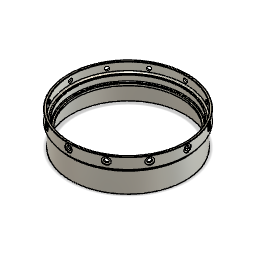
Connection-Ring-female-21.10.2024 v13 (Autodesk Fusion 360 design; units mm, degrees)
Autodesk Fusion 360 part; units mm, degrees
sketch "Skizze1" plane through (0, 0, 0) normal (0, 0, 1) x (1, 0, 0)
  line L0 (-83, 47) -> (-83, 30)
  line L1 (-83, 30) -> (-80, 30)
  line L2 (-80, 30) -> (-80, 0)
  line L3 (-73, 22.5) -> (-73, 25.5)
  line L4 (-73, 25.5) -> (-76, 25.5)
  line L5 (-76, 25.5) -> (-76, 34)
  line L6 (-76, 34) -> (-80, 34)
  line L7 (-80, 34) -> (-80, 47)
  line L8 (-80, 47) -> (-83, 47)
  line L9 (-80, 0) -> (-79, 0)
  line L10 (-76.75, 22.5) -> (-73, 22.5)
  line L11 (-76.75, 22.5) -> (-79, 0)
  line L12 (-76, 30) -> (-76.75, 22.5)
  dimension "d2" = 3
  dimension "d6" = 13
  dimension "d7" = 80
  dimension "d8" = 3
  dimension "d9" = 4
  dimension "d10" = 3
  dimension "d21" = 4
  dimension "d22" = 8.5
  dimension "d23" = 3
  dimension "d24" = 30
  dimension "d25" = 1
  constraint vertical L0
  constraint perpendicular L0 L1
  constraint perpendicular L1 L2
  constraint perpendicular L2 L4
  constraint perpendicular L5 L6
  constraint perpendicular L6 L7
  constraint perpendicular L0 L8
  constraint perpendicular L2 L9
  constraint horizontal origin L2.end
  constraint coincident L5 L12.start
  constraint collinear L11 L12
  constraint horizontal L1.end L12.start
  measures "d2" distance of L3 L5
  measures "d6" distance of L6 L8
  measures "d7" distance of origin L2
  measures "d8" distance of L0 L7
  measures "d9" distance of L2 L5
  measures "d10" distance of L0 L2
  measures "d21" distance of L1 L6
  measures "d22" distance of L4 L6
  measures "d23" distance of L4 L10
  measures "d24" distance of L1 L9
  measures "d25" distance of L2.end L9.end
revolve "Drehen1" add sketch "Skizze1" angle 360 about axis through (0, 1.75, 0) along (0, 1, 0)
fillet "Abrundung1" radius 2 1 edges at (-77.3832, 30, 30.0141)
fillet "Abrundung2" radius 2 1 edges at (-74.5862, 30, 28.9292)
fillet "Abrundung3" radius 2 1 edges at (-74.5862, 34, 28.9292)
chamfer "Fase3" distance 1 angle 45 1 edges at (-70.8569, 25.5, 27.4828)
ref_plane "Arbeitsebene1" through (83, 38.5, 0) normal (1, 0, 0) x (0, 0, -1)
sketch "Skizze4" plane through (83, 0, 0) normal (1, 0, 0) x (0, 0, -1)
  line L0 (-82.5, 47) -> (82.5, 47)
  point P0 (0, 40.5)
  dimension "d34" = 6.5
  constraint vertical origin P0
  measures "d34" distance of P0 L0
hole "Bohrung2" at (83, 40.5, 0) direction (-1, 0, 0) diameter 5.5 depth 16 tip angle 118 counterbore diameter 10 counterbore depth 1
pattern_circular "C-Anordnung1" count 12 over 360 about axis through (0, 1.75, 0) along (0, 1, 0) of "Bohrung2"
chamfer "Fase4" distance 0.4 angle 45 7 edges at (-74.5862, 47, 28.9292) (-70.8569, 34, 27.4828) (-74.5862, 0, 28.9292) (-73.6539, 0, 28.5676) (-71.5561, 22.5, 27.754) (-68.0599, 22.5, 26.3979) (-77.3832, 47, 30.0141)
equation "d7 = ( 160 / 2 ) * 1 mm"
equation "d22 = 15 mm - d6 / 2"
